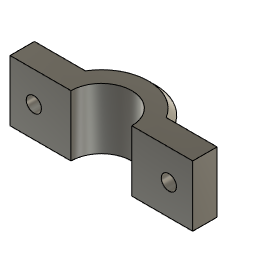
cable holder v1 (Autodesk Fusion 360 design; units mm, degrees)
Autodesk Fusion 360 part; units mm, degrees
sketch "Sketch1" plane through (0, 0, 0) normal (0, 0, 1) x (1, 0, 0)
  line L0 (-10, 0) -> (-30, 0)
  line L1 (10, 0) -> (30, 0)
  line L2 (-30, 0) -> (-30, 10)
  line L3 (30, 0) -> (30, 10)
  arc A0 (14.3614, 10) -> (-14.3614, 10) centre (0, 0) ccw
  line L4 (-30, 10) -> (-14.3614, 10)
  line L5 (14.3614, 10) -> (30, 10)
  arc A1 (10, 0) -> (-10, 0) centre (0, 0) ccw
  dimension "d1" = 20
  dimension "d2" = 35
  constraint coincident A0.centre A1.centre
  constraint horizontal L0
  constraint parallel L0 L1
  constraint perpendicular L0 L2
  constraint perpendicular L2 L4
  constraint perpendicular L3 L4
  constraint collinear L4 L5
  measures "d1" diameter of A1
  measures "d2" diameter of A0
extrude "Extrude1" add sketch "Sketch1" along normal blind 20
sketch "Sketch2" plane through (0, 10, 0) normal (0, 1, 0) x (-1, 0, 0)
  line L0 (-30, 0) -> (-14.3614, 0)
  line L1 (-14.3614, 0) -> (-14.3614, 20)
  line L2 (-14.3614, 20) -> (-30, 20)
  line L3 (-30, 20) -> (-30, 0)
  line L4 (-30, 20) -> (-14.3614, 0)
  line L5 (-14.3614, 20) -> (-30, 0)
  constraint coincident L2.end L3.start
  constraint coincident L0.end L1.start
  constraint coincident L1.end L2.start
  constraint coincident L0.start L3.end
hole "Hole1" at (22.1807, 10, 10) direction (0, -1, 0) diameter 5 depth 10 tip angle 118 countersink diameter 10 countersink angle 90
sketch "Sketch3" plane through (0, 10, 0) normal (0, 1, 0) x (-1, 0, 0)
  line L0 (14.3614, 0) -> (30, 0)
  line L1 (30, 0) -> (30, 20)
  line L2 (30, 20) -> (14.3614, 20)
  line L3 (14.3614, 20) -> (14.3614, 0)
  line L4 (14.3614, 20) -> (30, 0)
  line L5 (14.3614, 0) -> (30, 20)
  constraint coincident L2.end L3.start
  constraint coincident L0.end L1.start
  constraint coincident L0.start L3.end
  constraint coincident L1.end L2.start
hole "Hole2" at (-22.1807, 10, 10) direction (0, -1, 0) diameter 5 depth 10 tip angle 118 countersink diameter 10 countersink angle 90
chamfer "Chamfer1" distance 2 angle 45 8 edges at (-30, 10, 10) (30, 10, 10) (22.1807, 10, 0) (-22.1807, 10, 0) (-22.1807, 10, 20) (22.1807, 10, 20) (0, 17.5, 20) (0, 17.5, 0)
